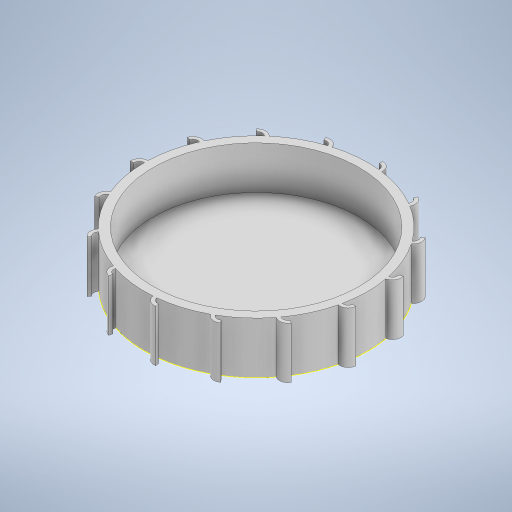
# Autodesk Inventor part: wheel_rib_ant1
Saved by Autodesk Inventor 2023 (Build 270158000, 158)
## iProperties
Created: 2022-10-08
Part Number: wheel_rib_ant1
Material: 一般
Document SubType Name: Modeling
Designer: Akio
Density: 1 g/cm^3
Appearance: 既定
Author: Akio
Autodesk Inventor part; units mm, degrees
ref_plane "YZ Plane" through (0, 0, 0) normal (1, 0, 0) x (0, 1, 0)
ref_plane "XZ Plane" through (0, 0, 0) normal (0, 1, 0) x (-1, 0, 0)
ref_plane "XY Plane" through (0, 0, 0) normal (0, 0, 1) x (1, 0, 0)
sketch "スケッチ1" plane through (0, 0, 0) normal (1, 0, 0) x (0, 1, 0)
  point P0 (0, 0)
sketch "スケッチ2" plane through (0, 0, 0) normal (0, 1, 0) x (-1, 0, 0)
  circle A0 centre (0, 0) radius 65
  dimension "d1" = 130
  constraints: 1 centre point, 1 coincident
  measures "d1" diameter of A0
extrude "押し出し1" add sketch "スケッチ2" along normal blind 30
sketch "スケッチ3" plane through (0, 30, 0) normal (0, 1, 0) x (1, 0, 0)
  circle A0 centre (0, 0) radius 60
  dimension "d4" = 120
  constraints: 1 centre point, 1 coincident
  measures "d4" diameter of A0
extrude "押し出し2" cut sketch "スケッチ3" against normal blind 25
sketch "スケッチ4" plane through (0, 0, 0) normal (0, -1, 0) x (1, 0, 0)
  circle A0 centre (0, 0) radius 65 projected
  arc A1 (-64.9694, -1.9949) -> (-61.7673, -0.8673) centre (-64.9305, 3.005) ccw
  arc A2 (-69.9053, 3.5064) -> (-61.7673, -0.8673) centre (-64.9305, 3.005) ccw
  line L0 (-64.9305, 3.005) -> (-69.9053, 3.5064) construction
  line L1 (-64.9305, 3.005) -> (-61.7673, -0.8673) construction
  arc A3 (-67.9154, 3.3058) -> (-64.6802, 0.0154) centre (-64.9305, 3.005) ccw
  line L2 (-69.9053, 3.5064) -> (-67.9154, 3.3058)
  line L3 (-60.5392, -23.6644) -> (-65.2878, -25.2298) construction
  arc A4 (-63.3884, -24.6037) -> (-59.0946, -26.2937) centre (-60.5392, -23.6644) ccw
  arc A5 (-65.2878, -25.2298) -> (-56.0745, -25.9153) centre (-60.5392, -23.6644) ccw
  line L4 (-65.2878, -25.2298) -> (-63.3884, -24.6037)
  line L5 (-45.6801, -46.242) -> (-49.3815, -49.6035) construction
  arc A6 (-47.901, -48.2589) -> (-43.291, -48.0565) centre (-45.6801, -46.242) ccw
  arc A7 (-49.3815, -49.6035) -> (-40.6859, -46.4824) centre (-45.6801, -46.242) ccw
  line L6 (-49.3815, -49.6035) -> (-47.901, -48.2589)
  line L7 (-22.9225, -60.824) -> (-24.9367, -65.4004) construction
  arc A8 (-24.131, -63.5698) -> (-20.002, -61.5098) centre (-22.9225, -60.824) ccw
  arc A9 (-24.9367, -65.4004) -> (-18.2623, -59.0122) centre (-22.9225, -60.824) ccw
  line L8 (-24.9367, -65.4004) -> (-24.131, -63.5698)
  line L9 (3.7986, -64.8889) -> (3.8199, -69.8889) construction
  arc A10 (3.8114, -67.8889) -> (6.7456, -64.3275) centre (3.7986, -64.8889) ccw
  arc A11 (3.8199, -69.8889) -> (7.319, -61.3383) centre (3.7986, -64.8889) ccw
  line L10 (3.8199, -69.8889) -> (3.8114, -67.8889)
  line L11 (29.8629, -57.734) -> (31.916, -62.293) construction
  arc A12 (31.0948, -60.4694) -> (32.3267, -56.0225) centre (29.8629, -57.734) ccw
  arc A13 (31.916, -62.293) -> (31.6347, -53.0584) centre (29.8629, -57.734) ccw
  line L12 (31.916, -62.293) -> (31.0948, -60.4694)
  line L13 (50.7636, -40.5963) -> (54.4936, -43.926) construction
  arc A14 (53.0016, -42.5941) -> (52.3183, -38.0306) centre (50.7636, -40.5963) ccw
  arc A15 (54.4936, -43.926) -> (50.4806, -35.6043) centre (50.7636, -40.5963) ccw
  line L14 (54.4936, -43.926) -> (53.0016, -42.5941)
  line L15 (62.8868, -16.4391) -> (67.6487, -17.9639) construction
  arc A16 (65.7439, -17.354) -> (63.2636, -13.4629) centre (62.8868, -16.4391) ccw
  arc A17 (67.6487, -17.9639) -> (60.5979, -11.9938) centre (62.8868, -16.4391) ccw
  line L16 (67.6487, -17.9639) -> (65.7439, -17.354)
  line L17 (64.1364, 10.5605) -> (69.1067, 11.1044) construction
  arc A18 (67.1186, 10.8868) -> (63.27, 13.4327) centre (64.1364, 10.5605) ccw
  arc A19 (69.1067, 11.1044) -> (60.2372, 13.6905) centre (64.1364, 10.5605) ccw
  line L18 (69.1067, 11.1044) -> (67.1186, 10.8868)
  line L19 (54.2962, 35.7341) -> (58.6156, 38.2526) construction
  arc A20 (56.8878, 37.2452) -> (52.3365, 38.0056) centre (54.2962, 35.7341) ccw
  arc A21 (58.6156, 38.2526) -> (49.4611, 37.0076) centre (54.2962, 35.7341) ccw
  line L20 (58.6156, 38.2526) -> (56.8878, 37.2452)
  line L21 (35.0676, 54.729) -> (37.9893, 58.7866) construction
  arc A22 (36.8206, 57.1635) -> (32.3535, 56.007) centre (35.0676, 54.729) ccw
  arc A23 (37.9893, 58.7866) -> (30.1326, 53.9257) centre (35.0676, 54.729) ccw
  line L22 (37.9893, 58.7866) -> (36.8206, 57.1635)
  line L23 (9.7756, 64.2607) -> (10.7943, 69.1558) construction
  arc A24 (10.3868, 67.1978) -> (6.7763, 64.3243) centre (9.7756, 64.2607) ccw
  arc A25 (10.7943, 69.1558) -> (5.5939, 61.5196) centre (9.7756, 64.2607) ccw
  line L24 (10.7943, 69.1558) -> (10.3868, 67.1978)
  line L25 (-17.2067, 62.6812) -> (-18.2672, 67.5674) construction
  arc A26 (-17.843, 65.6129) -> (-19.9726, 61.5193) centre (-17.2067, 62.6812) ccw
  arc A27 (-18.2672, 67.5674) -> (-19.912, 58.4762) centre (-17.2067, 62.6812) ccw
  line L26 (-18.2672, 67.5674) -> (-17.843, 65.6129)
  line L27 (-41.2138, 50.2635) -> (-44.17, 54.296) construction
  arc A28 (-42.9876, 52.683) -> (-43.268, 48.0771) centre (-41.2138, 50.2635) ccw
  arc A29 (-44.17, 54.296) -> (-41.9749, 45.3218) centre (-41.2138, 50.2635) ccw
  line L28 (-44.17, 54.296) -> (-42.9876, 52.683)
  line L29 (-58.0947, 29.1548) -> (-62.4355, 31.6363) construction
  arc A30 (-60.6992, 30.6437) -> (-59.0821, 26.3219) centre (-58.0947, 29.1548) ccw
  arc A31 (-62.4355, 31.6363) -> (-56.78, 24.3308) centre (-58.0947, 29.1548) ccw
  line L30 (-62.4355, 31.6363) -> (-60.6992, 30.6437)
  point P0 (-21.9739, 61.1731)
  point P1 (-20.0806, 61.8205)
  point P2 (4.8072, 64.822)
  point P3 (6.8001, 64.6433)
  point P4 (30.7571, 57.2626)
  point P5 (32.505, 56.2888)
  point P6 (51.3888, 39.8019)
  point P7 (52.5895, 38.2014)
  point P8 (63.1349, 15.4592)
  point P9 (63.5808, 13.5086)
  point P10 (63.9644, -11.5566)
  point P11 (63.5784, -13.5199)
  point P12 (53.7339, -36.5742)
  point P13 (52.5827, -38.2107)
  point P14 (34.2123, -55.2677)
  point P15 (32.495, -56.2945)
  point P16 (8.7751, -64.405)
  point P17 (6.7886, -64.6445)
  point P18 (-18.1794, -62.406)
  point P19 (-20.0916, -61.8169)
  point P20 (-41.9905, -49.6165)
  point P21 (-43.4978, -48.3005)
  point P22 (-58.5411, -28.2478)
  point P23 (-59.3828, -26.4326)
  point P24 (-44.9555, 46.9468)
  point P25 (-43.4892, 48.3083)
  point P26 (-60.1639, 24.603)
  point P27 (-59.3781, 26.4432)
  point P28 (-64.9694, -1.9949)
  point P29 (-65, 0.0058)
  dimension "d8" = 5
  dimension "d9" = 135
  dimension "d10" = 3
  dimension "d13" = 360
  constraints: 62 end point, 62 point on circle, 31 centre point, 16 coincident, 15 point on line, 154 other
  measures "d8" radius of A2
  measures "d9" angle of L0 L1
  measures "d10" radius of A3
sketch "スケッチ5" plane through (0, 0, 0) normal (0, -1, 0) x (1, 0, 0)
  circle A0 centre (0, 0) radius 65 projected
  line L0 (-65, 0) -> (-64.9694, -1.9932)
  constraints: 2 end point, 2 point on circle
sketch "スケッチ6" plane through (0, 0, 0) normal (0, -1, 0) x (1, 0, 0)
  point P0 (0, 0)
extrude "押し出し3" add sketch "スケッチ4" against normal blind 30 contours A0 A19 L18 A18 | A17 L16 A16 A0 | A0 A21 L20 A20 | A15 L14 A14 A0 | A0 A23 L22 A22 | A13 L12 A12 A0 | A0 A25 L24 A24 | A11 L10 A10 A0 | A0 A27 L26 A26 | A9 L8 A8 A0 | A0 A29 L28 A28 | A7 L6 A6 A0 | A0 A31 L30 A30 | A5 L4 A4 A0 | A0 A2 L2 A3
